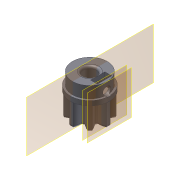
# Autodesk Inventor part: Engranaje_motor_Z
Saved by Autodesk Inventor 2015 SP2 (Build 190223200, 223)
## iProperties
Created: 2015-05-13
Material: Steel
Document SubType Name: Modeling
Designer: E.Beroiz
Categories: <?xml version="1.0" encoding="UTF-16"?> <MemberInstance><Categories><FamilyTemplate><FamilyTemplateParameter ValueType="xs:double" Id="1" ObjectReferenceKey="da_z" ObjectType="kUserParameterObject"/><FamilyTemplateParameter ValueType="xs:double" Id="2" ObjectReferenceKey="da_b" ObjectType="kUserParameterObject"/><FamilyTemplateParameter ValueType="xs:double" Id="3" ObjectReferenceKey="da_beta" ObjectType="kUserParameterObject"/><FamilyTemplateParameter ValueType="xs:double" Id="4" ObjectReferenceKey="da_da" ObjectType="kUserParameterObject"/><FamilyTemplateParameter ValueType="xs:double" Id="5" ObjectReferenceKey="da_aw" ObjectType="kUserParameterObject"/><FamilyTemplateParameter ValueType="xs:string" Id="6" ObjectReferenceKey="EAIAABAAAACIAQAAAAAAAIAAAAAAAAAA" ObjectType="83910656" SubObjectId="SurfaceGeometry"/></FamilyTemplate><ParamToTemplateMap><ParamToTemplate CategoryParameter="//CategoryParameter[@InternalName='046C89C9-8512-4d59-83FE-43B91F4F132A']" TemplateParameter="1"/><ParamToTemplate CategoryParameter="//CategoryParameter[@InternalName='2552DF32-E462-4b46-AEBF-C6C7768E72AC']" TemplateParameter="2"/><ParamToTemplate CategoryParameter="//CategoryParameter[@InternalName='C9EE641D-15FC-4fae-A226-E94C4372FDD7']" TemplateParameter="3"/><ParamToTemplate><ParamToTemplate CategoryParameter="//CategoryParameter[@InternalName='00B6519A-459B-49c7-AD84-2E56D39A5744']" ConstantValue="0.000000"/></ParamToTemplate><ParamToTemplate><ParamToTemplate CategoryParameter="//CategoryParameter[@InternalName='04B31F0E-C7A6-4894-AA32-9629BEFACF47']" ConstantValue="0.800000"/></ParamToTemplate><ParamToTemplate><ParamToTemplate CategoryParameter="//CategoryParameter[@InternalName='43CBEC2E-7847-49e7-A936-2F7889FCB2D9']" ConstantValue="0.300000"/></ParamToTemplate><ParamToTemplate><ParamToTemplate CategoryParameter="//CategoryParameter[@InternalName='B1EFC894-105D-4ebd-86BF-FA20ED196853']" ConstantValue="0.151900"/></ParamToTemplate><ParamToTemplate><ParamToTemplate CategoryParameter="//CategoryParameter[@InternalName='51175063-3D10-4879-93E8-6246FE8B403D']" ConstantValue="2060000000.000000"/></ParamToTemplate><ParamToTemplate><ParamToTemplate CategoryParameter="//CategoryParameter[@InternalName='A3A52E27-4454-46a9-B0BD-C932399B70AF']" ConstantValue="0.300000"/></ParamToTemplate><ParamToTemplate><ParamToTemplate CategoryParameter="//CategoryParameter[@InternalName='91B76062-C214-41d9-B1B9-14D2AB99603D']" ConstantValue="0.175000"/></ParamToTemplate><ParamToTemplate><ParamToTemplate CategoryParameter="//CategoryParameter[@InternalName='374E806E-8B8A-4dda-A9AA-1039D6500AD2']" ConstantValue="5.714286"/></ParamToTemplate><ParamToTemplate><ParamToTemplate CategoryParameter="//CategoryParameter[@InternalName='2D373A89-B862-43d6-8D0B-0CBF12AB9F6C']" ConstantValue="0.349066"/></ParamToTemplate><ParamToTemplate CategoryParameter="//CategoryParameter[@InternalName='37777632-D6A2-4fac-9D53-DB8ACD95C989']" TemplateParameter="4"/><ParamToTemplate CategoryParameter="//CategoryParameter[@InternalName='FD1017F1-B727-4f7e-9707-0F86F1FF9423']" TemplateParameter="5"/><ParamToTemplate><ParamToTemplate CategoryParameter="//CategoryParameter[@InternalName='9E1B4470-B2D3-4ff1-B813-535BB4CDF51A']" ConstantValue="3520000.000000"/></ParamToTemplate><ParamToTemplate><ParamToTemplate CategoryParameter="//CategoryParameter[@InternalName='F8452263-BFF6-458c-9FB1-07C4B99E95CD']" ConstantValue="11400000.000000"/></ParamToTemplate><ParamToTemplate><ParamToTemplate CategoryParameter="//CategoryParameter[@InternalName='3E3BB259-FD49-497f-8171-6EBC954A3479']" ConstantValue="2.000000"/></ParamToTemplate><ParamToTemplate CategoryParameter="//CategoryParameter[@InternalName='27C3BAF2-7550-4e4b-AE2C-0DB134B7D9B7']" TemplateParameter="6"/></ParamToTemplateMap><Category DisplayName="Gear" InternalName="DC85795E-93AB-48d5-8EEE-5A27447B64BD" Mnemonic="Gear"><CategoryParameter DisplayName="z" InternalName="046C89C9-8512-4d59-83FE-43B91F4F132A" Mnemonic="z"/><CategoryParameter DisplayName="b" InternalName="2552DF32-E462-4b46-AEBF-C6C7768E72AC" Mnemonic="b"/><CategoryParameter DisplayName="||b|" InternalName="C9EE641D-15FC-4fae-A226-E94C4372FDD7" Mnemonic="beta"/><CategoryParameter DisplayName="x" InternalName="00B6519A-459B-49c7-AD84-2E56D39A5744" Mnemonic="x"/><CategoryParameter DisplayName="a*" InternalName="04B31F0E-C7A6-4894-AA32-9629BEFACF47" Mnemonic="a"/><CategoryParameter DisplayName="c*" InternalName="43CBEC2E-7847-49e7-A936-2F7889FCB2D9" Mnemonic="c"/><CategoryParameter DisplayName="r|.f|*" InternalName="B1EFC894-105D-4ebd-86BF-FA20ED196853" Mnemonic="rf"/><CategoryParameter DisplayName="E" InternalName="51175063-3D10-4879-93E8-6246FE8B403D" Mnemonic="E"/><CategoryParameter DisplayName="||m|" InternalName="A3A52E27-4454-46a9-B0BD-C932399B70AF" Mnemonic="mi"/><Category DisplayName="SpurGear" InternalName="26C5A22E-A91E-4dfd-A3B3-23CCAFAE1764" Mnemonic="SpurGear"><CategoryParameter DisplayName="m" InternalName="91B76062-C214-41d9-B1B9-14D2AB99603D" Mnemonic="m"/><CategoryParameter DisplayName="P" InternalName="374E806E-8B8A-4dda-A9AA-1039D6500AD2" Mnemonic="PP"/><CategoryParameter DisplayName="||a|" InternalName="2D373A89-B862-43d6-8D0B-0CBF12AB9F6C" Mnemonic="alpha"/><CategoryParameter DisplayName="d|.a|" InternalName="37777632-D6A2-4fac-9D53-DB8ACD95C989" Mnemonic="da"/><CategoryParameter DisplayName="a|.w|" InternalName="FD1017F1-B727-4f7e-9707-0F86F1FF9423" Mnemonic="aw"/><CategoryParameter DisplayName="||s||.Flim|" InternalName="9E1B4470-B2D3-4ff1-B813-535BB4CDF51A" Mnemonic="sFlim"/><CategoryParameter DisplayName="||s||.Hlim|" InternalName="F8452263-BFF6-458c-9FB1-07C4B99E95CD" Mnemonic="sHlim"/><CategoryParameter DisplayName="tipo" InternalName="3E3BB259-FD49-497f-8171-6EBC954A3479" Mnemonic="type"/><CategoryParameter DisplayName="PitchDiameter" InternalName="27C3BAF2-7550-4e4b-AE2C-0DB134B7D9B7" Mnemonic="IDS_PITCHDIAM"/></Category></Category></Categories></MemberInstance>
Density: 1 g/cm^3
Appearance: Steel
Description: Cycl_enganajeMotorZ
CustomPartVersion: 1
Author: E.Beroiz
Autodesk Inventor part; units mm, degrees
ref_plane "XZ Plane" through (0, 0, 0) normal (0, 1, 0) x (-1, 0, 0)
sketch "Sketch1" plane through (0, 0, 0) normal (0, 0, 1) x (1, 0, 0)
  circle A0 centre (0, 0) radius 8.0433
  dimension "d0" = 16.0865
  constraints: 1 centre point
  measures "d0" diameter of A0
extrude "Extrusion1" add sketch "Sketch1" along normal blind 10
ref_plane "Work Plane2" through (0, 0, 5) normal (0, 0, 1) x (1, 0, 0)
sketch "Sketch2" plane through (0, 0, 0) normal (0, 0, -1) x (-1, 0, 0)
  circle A0 centre (0, 0) radius 8.0433 projected
  circle A1 centre (0, 0) radius 6.6087
  dimension "d3" = 13.2174
  constraints: 1 centre point, 1 coincident
  measures "d3" diameter of A1
surface extrude "Diámetro de separación" sketch "Sketch2" against normal through all shown no curves A1
ref_plane "Work Plane8" through (0, 0, 0) normal (0.9238795, 0.3826834, 0) x (0, 0, 1)
ref_plane "Work Plane9" through (0, 0, 0) normal (1, 0, 0) x (0, 1, 0)
spur gear teeth "Engranaje recto" teeth 8 pitch diameter 14 tip diameter 16.0865 root diameter 10.15 face width 10 start plane through (0, 0, 0) normal (0, 0, -1) x (-1, 0, 0)
sketch "Boceto6" plane through (0, 0, 10) normal (0, 0, 1) x (1, 0, 0)
  circle A0 centre (0, 0) radius 8.4
  dimension "d55" = 16.8
  constraints: 1 centre point, 1 coincident
  measures "d55" diameter of A0
extrude "Extrusión4" add sketch "Boceto6" along normal blind 7
hole "Agujero1" at (0, 0, 17) direction (0, 0, -1) diameter 5.7 end through all
ref_plane "Plano de trabajo11" through (8.4, 0, 10) normal (1, 0, 0) x (0, 1, 0)
sketch "Boceto7" plane through (8.4, 0, 10) normal (1, 0, 0) x (0, 1, 0)
  line L0 (8.4, 7) -> (-8.4, 7) projected
  line L1 (-8.4, 0) -> (8.4, 0) projected
  circle A0 centre (0, 3.5) radius 1.725
  line L2 (-8.4, 0) -> (-8.4, 7) projected
  point P0 (0, -10)
  point P1 (-8.75, 0)
  point P2 (8.75, 0)
  point P3 (0, 7)
  point P4 (-8.4, 3.5)
  dimension "d67" = 3.45
  constraints: 1 centre point, 1 horizontal alignment, 1 midpoint, 1 vertical alignment, 2 other
  measures "d67" diameter of A0
extrude "Extrusión5" cut sketch "Boceto7" against normal up to surface round surface about axis through (0, 0, -12.2144) along (0, 0, 1) radius 2.85 far side no
ref_plane "Plano de trabajo12" through (6.4, 0, 10) normal (1, 0, 0) x (0, 1, 0)
sketch "Boceto8" plane through (6.4, 0, 10) normal (1, 0, 0) x (0, 1, 0)
  line L0 (-8.0045, 0) -> (-4.8565, 0) projected
  line L1 (-8.0045, -10) -> (-8.0045, 0) projected
  line L2 (-4.8565, -10) -> (-8.0045, -10) projected
  line L3 (-4.8565, -10) -> (-4.8565, 0) projected
  spline S0 degree 2 poles (1.725, 3.5) (1.725, 6.4878) (-0.8625, 4.9939) (-3.45, 3.5) (-0.8625, 2.0061) (1.725, 0.5122) (1.725, 3.5) knots 0 0 0 0.333333 0.333333 0.666667 0.666667 1 1 1 weights 1 0.5 1 0.5 1 0.5 1 projected
  line L4 (0, 7.0796) -> (3.1, 5.2898)
  line L5 (3.1, 5.2898) -> (3.1, 1.7102)
  line L6 (3.1, 1.7102) -> (0, -0.0796)
  line L7 (0, -0.0796) -> (-3.1, 1.7102)
  line L8 (-3.1, 1.7102) -> (-3.1, 5.2898)
  line L9 (2.85, -10) -> (-2.85, -10) projected
  line L10 (-2.85, 7) -> (2.85, 7) projected
  line L11 (8.4, 0) -> (8.4, 7) projected
  line L12 (-3.1, 5.2898) -> (-3.1, 7.2898)
  line L13 (-3.1, 7.2898) -> (3.1, 7.2898)
  line L14 (3.1, 7.2898) -> (3.1, 5.2898)
  point P0 (0, -10)
  point P1 (0, 3.5)
  point P2 (0, 7)
  point P3 (8.4, 3.5)
  dimension "d71" = 6.2
  dimension "d72" = 2
  constraints: 16 end point, 2 midpoint, 2 perpendicular, 2 vertical alignment, 1 horizontal alignment, 1 vertical, 13 other
  measures "d71" distance between parallel lines of L8 L5
  measures "d72" distance of L13.end L4.end
extrude "Extrusión6" cut sketch "Boceto8" against normal blind 3 contours L5 L6 L7 L8 L12 L13 L14
fillet "Empalme1" radius 1 1 edges at (0, 2.85, 17)
fillet "Empalme2" radius 1 32 edges at (-5.5258, 3.6323, 0) (-5.6874, 5.6874, 0) (-3.6323, 5.5258, 0) (-1.9421, 4.6887, 0) (-1.3389, 6.4758, 0) (0, 8.0433, 0) (1.3389, 6.4758, 0) (1.9421, 4.6887, 0) (3.6323, 5.5258, 0) (5.6874, 5.6874, 0) (5.5258, 3.6323, 0) (4.6887, 1.9421, 0) (6.4758, 1.3389, 0) (8.0433, 0, 0) (6.4758, -1.3389, 0) (4.6887, -1.9421, 0) (5.5258, -3.6323, 0) (5.6874, -5.6874, 0) (3.6323, -5.5258, 0) (1.9421, -4.6887, 0) (1.3389, -6.4758, 0) (0, -8.0433, 0) (-1.3389, -6.4758, 0) (-1.9421, -4.6887, 0) (-3.6323, -5.5258, 0) (-5.6874, -5.6874, 0) (-5.5258, -3.6323, 0) (-4.6887, -1.9421, 0) (-6.4758, -1.3389, 0) (-8.0433, 0, 0) (-6.4758, 1.3389, 0) (-4.6887, 1.9421, 0)
sketch "Boceto9" plane through (0, 0, 17) normal (0, 0, 1) x (1, 0, 0)
  circle A0 centre (0, 0) radius 7.5
  line L0 (-19.4241, -19.0827) -> (-22.6844, 15.062) projected
  line L1 (-19.4241, -19.0827) -> (-15.062, -22.6844) projected
  line L2 (-6.1028, -21.8289) -> (-15.062, -22.6844) projected
  line L3 (-6.1028, -21.8289) -> (-5.7226, -25.8108) projected
  line L4 (-5.7226, -25.8108) -> (10.5036, -24.2615) projected
  line L5 (10.5036, -24.2615) -> (10.1234, -20.2796) projected
  line L6 (19.0827, -19.4241) -> (10.1234, -20.2796) projected
  line L7 (19.0827, -19.4241) -> (22.6844, -15.062) projected
  line L8 (19.4241, 19.0827) -> (22.6844, -15.062) projected
  line L9 (19.4241, 19.0827) -> (15.062, 22.6844) projected
  line L10 (-19.0827, 19.4241) -> (15.062, 22.6844) projected
  line L11 (-19.0827, 19.4241) -> (-22.6844, 15.062) projected
  circle A1 centre (13.9565, 16.9031) radius 1.5 projected
  circle A2 centre (-16.9031, 13.9565) radius 1.5 projected
  circle A3 centre (-13.9565, -16.9031) radius 1.5 projected
  circle A4 centre (0, 0) radius 4.5 projected
  circle A5 centre (16.9031, -13.9565) radius 1.5 projected
  circle A6 centre (0, 0) radius 8.4 projected
  dimension "d82" = 15
  constraints: 1 centre point, 1 coincident
  measures "d82" diameter of A0
extrude "Extrusión7" cut sketch "Boceto9" against normal blind 5 contours A6
equation "\"d0\" = da_da"
equation "\"d1\" = da_b"
equation "\"d3\" = da_dw"
equation "\"d16\" = da_aw"
equation "\"d43\" = da_aw"
equation "\"d46\" = da_aw"
equation "\"da_da\" = 16.0865"
equation "\"da_b\" = 10"
equation "\"da_dw\" = 13.217391"
equation "\"da_aw\" = 19"
body "Solid1"
body "Srf1"
